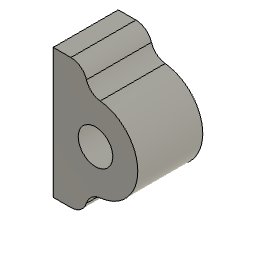
magnet_mount (Autodesk Fusion 360 design; units mm, degrees)
Autodesk Fusion 360 part; units mm, degrees
note: some values were not read from the file. Set by a fixed rule: which sketch regions a step uses.
sketch "Sketch1" plane through (0, 0, 0) normal (0, 1, 0) x (1, 0, 0)
  circle A0 centre (0, 0) radius 3.175
  circle A1 centre (0, 0) radius 8.255
  line L0 (-1.905, -12.7) -> (-8.255, -12.7)
  line L1 (-8.255, -12.7) -> (-8.255, 12.7)
  line L2 (-8.255, 12.7) -> (-1.905, 12.7)
  line L3 (-1.905, 12.7) -> (-1.905, -12.7)
  circle A2 centre (1.27, -11.3592) radius 3.175
  circle A3 centre (1.27, 11.3592) radius 3.175
  circle A4 centre (0, 0) radius 3.375
  point P0 (-8.255, 0)
  dimension "d1" = 6.35
  dimension "d2" = 5.08
  dimension "d3" = 6.35
  dimension "d4" = 25.4
  dimension "d5" = 6.35
  dimension "d10" = 0.2
  constraint coincident A0.centre A1.centre
  constraint concentric A0 A1
  constraint horizontal L0
  constraint vertical L1
  constraint horizontal L2
  constraint vertical L3
  constraint midpoint L1 P0
  constraint horizontal A0.centre P0
  constraint tangent L3 A2
  constraint tangent A1 A2
  constraint equal A2 A3
  constraint tangent A1 A3
  constraint tangent L3 A3
  constraint tangent A1 L1
  measures "d1" diameter of A0
  measures "d2" distance of A0 A1
  measures "d3" distance of L0.start L0.end
  measures "d4" distance of L0 L2
  measures "d5" diameter of A2
  measures "d10" distance of A0 A4
extrude "Extrude1" add sketch "Sketch1" along normal blind 12.7 contours A0 L3 | A0 L3 A4 | A0 L3 | A0 L3 A4 | A1 L3 A4 | A1 L3 A4 | A1 L3 A3 | A1 L1 L2 L3 | A1 L0 L1 L3 | A1 L3 A2
extrude "Extrude2" cut sketch "Sketch1" along normal blind 6.35 contours A0 L3 | A0 L3 A4 | A0 L3 | A0 L3 A4
fillet "Fillet5" radius 3.175 2 edges at (-1.905, 6.35, -12.7) (-1.905, 6.35, 12.7)
